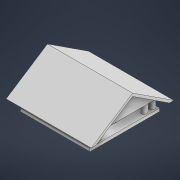
# Autodesk Inventor part: 110033226_ipt_15_房子屋頂
Saved by Autodesk Inventor 2022 (Build 260153000, 153)
## iProperties
Created: 2022-06-23
Part Number: 110033226_ipt_15_房子屋頂
Material: 一般
Document SubType Name: Modeling
Designer: User
Density: 1 g/cm^3
Appearance: 預設
Author: User
Autodesk Inventor part; units mm, degrees
ref_plane "YZ Plane" through (0, 0, 0) normal (1, 0, 0) x (0, 1, 0)
ref_plane "XZ Plane" through (0, 0, 0) normal (0, 1, 0) x (-1, 0, 0)
ref_plane "XY Plane" through (0, 0, 0) normal (0, 0, 1) x (1, 0, 0)
sketch "草圖1" plane through (0, 0, 0) normal (0, 1, 0) x (-1, 0, 0)
  line L0 (22.5, 22.5) -> (-22.5, 22.5)
  line L1 (-22.5, 22.5) -> (-22.5, -22.5)
  line L2 (-22.5, -22.5) -> (22.5, -22.5)
  line L3 (22.5, -22.5) -> (22.5, 22.5)
  circle A0 centre (20, 20) radius 1.7
  circle A1 centre (20, 15) radius 1.7
  circle A2 centre (20, 10) radius 1.7
  circle A3 centre (20, 5) radius 1.7
  circle A4 centre (20, 0) radius 1.7
  circle A5 centre (20, -5) radius 1.7
  circle A6 centre (20, -10) radius 1.7
  circle A7 centre (20, -15) radius 1.7
  circle A8 centre (20, -20) radius 1.7
  circle A9 centre (15, 20) radius 1.7
  circle A10 centre (15, 15) radius 1.7
  circle A11 centre (15, 10) radius 1.7
  circle A12 centre (15, 5) radius 1.7
  circle A13 centre (15, 0) radius 1.7
  circle A14 centre (15, -5) radius 1.7
  circle A15 centre (15, -10) radius 1.7
  circle A16 centre (15, -15) radius 1.7
  circle A17 centre (15, -20) radius 1.7
  circle A18 centre (10, 20) radius 1.7
  circle A19 centre (10, 15) radius 1.7
  circle A20 centre (10, 10) radius 1.7
  circle A21 centre (10, 5) radius 1.7
  circle A22 centre (10, 0) radius 1.7
  circle A23 centre (10, -5) radius 1.7
  circle A24 centre (10, -10) radius 1.7
  circle A25 centre (10, -15) radius 1.7
  circle A26 centre (10, -20) radius 1.7
  circle A27 centre (5, 20) radius 1.7
  circle A28 centre (5, 15) radius 1.7
  circle A29 centre (5, 10) radius 1.7
  circle A30 centre (5, 5) radius 1.7
  circle A31 centre (5, 0) radius 1.7
  circle A32 centre (5, -5) radius 1.7
  circle A33 centre (5, -10) radius 1.7
  circle A34 centre (5, -15) radius 1.7
  circle A35 centre (5, -20) radius 1.7
  circle A36 centre (0, 20) radius 1.7
  circle A37 centre (0, 15) radius 1.7
  circle A38 centre (0, 10) radius 1.7
  circle A39 centre (0, 5) radius 1.7
  circle A40 centre (0, 0) radius 1.7
  circle A41 centre (0, -5) radius 1.7
  circle A42 centre (0, -10) radius 1.7
  circle A43 centre (0, -15) radius 1.7
  circle A44 centre (0, -20) radius 1.7
  circle A45 centre (-5, 20) radius 1.7
  circle A46 centre (-5, 15) radius 1.7
  circle A47 centre (-5, 10) radius 1.7
  circle A48 centre (-5, 5) radius 1.7
  circle A49 centre (-5, 0) radius 1.7
  circle A50 centre (-5, -5) radius 1.7
  circle A51 centre (-5, -10) radius 1.7
  circle A52 centre (-5, -15) radius 1.7
  circle A53 centre (-5, -20) radius 1.7
  circle A54 centre (-10, 20) radius 1.7
  circle A55 centre (-10, 15) radius 1.7
  circle A56 centre (-10, 10) radius 1.7
  circle A57 centre (-10, 5) radius 1.7
  circle A58 centre (-10, 0) radius 1.7
  circle A59 centre (-10, -5) radius 1.7
  circle A60 centre (-10, -10) radius 1.7
  circle A61 centre (-10, -15) radius 1.7
  circle A62 centre (-10, -20) radius 1.7
  circle A63 centre (-15, 20) radius 1.7
  circle A64 centre (-15, 15) radius 1.7
  circle A65 centre (-15, 10) radius 1.7
  circle A66 centre (-15, 5) radius 1.7
  circle A67 centre (-15, 0) radius 1.7
  circle A68 centre (-15, -5) radius 1.7
  circle A69 centre (-15, -10) radius 1.7
  circle A70 centre (-15, -15) radius 1.7
  circle A71 centre (-15, -20) radius 1.7
  circle A72 centre (-20, 20) radius 1.7
  circle A73 centre (-20, 15) radius 1.7
  circle A74 centre (-20, 10) radius 1.7
  circle A75 centre (-20, 5) radius 1.7
  circle A76 centre (-20, 0) radius 1.7
  circle A77 centre (-20, -5) radius 1.7
  circle A78 centre (-20, -10) radius 1.7
  circle A79 centre (-20, -15) radius 1.7
  circle A80 centre (-20, -20) radius 1.7
  point P0 (0, 0)
  point P1 (22.5, 0)
  point P2 (0, -22.5)
  dimension "d0" = 45
  dimension "d1" = 45
  dimension "d2" = 3.4
  dimension "d3" = 2.5
  dimension "d4" = 2.5
  dimension "d7" = 5
  dimension "d10" = 5
  constraints: 81 centre point, 8 end point, 2 horizontal, 2 midpoint, 2 parallel, 1 horizontal alignment, 1 perpendicular, 1 vertical, 1 vertical alignment, 160 other
  measures "d0" distance of L2.end L1.end
  measures "d1" distance of L1.end L0.end
  measures "d2" diameter of A0
  measures "d3" distance from line of L3 A0.centre
  measures "d4" distance from line of L0 A0.centre
  measures "d7" distance of A0.centre A1.centre
  measures "d10" distance of A0.centre A9.centre
extrude "擠出1" add sketch "草圖1" along normal blind 6 contours A0 | A1 | A7 | A8 | A9 | A13 | A17 | A36 | A37 | A43 | A44 | A63 | A67 | A71 | A72 | A73 | A79 | A80
extrude "擠出2" add sketch "草圖1" against normal blind 2 contours L3 L2 L1 L0 | A0 | A1 | A2 | A3 | A4 | A5 | A6 | A7 | A8 | A9 | A10 | A11 | A12 | A13 | A14 | A15 | A16 | A17 | A18 | A19 | A20 | A21 | A22 | A23 | A24 | A25 | A26 | A27 | A28 | A29 | A30 | A31 | A32 | A33 | A34 | A35 | A36 | A37 | A38 | A39 | A40 | A41 | A42 | A43 | A44 | A45 | A46 | A47 | A48 | A49 | A50 | A51 | A52 | A53 | A54 | A55 | A56 | A57 | A58 | A59 | A60 | A61 | A62 | A63 | A64 | A65 | A66 | A67 | A68 | A69 | A70 | A71 | A72 | A73 | A74 | A75 | A76 | A77 | A78 | A79 | A80
sketch "草圖2" plane through (0, -2, 0) normal (0, -1, 0) x (1, 0, 0)
  circle A0 centre (20, 20) radius 1.7 projected
  circle A1 centre (20, 15) radius 1.7 projected
  circle A2 centre (15, 20) radius 1.7 projected
  line L0 (22.5, 22.5) -> (22.5, -22.5) projected
  line L1 (22.5, -22.5) -> (-22.5, -22.5) projected
  line L2 (-22.5, -22.5) -> (-22.5, 22.5) projected
  line L3 (-22.5, 22.5) -> (22.5, 22.5) projected
  circle A3 centre (20, 20) radius 1.7 projected
  circle A4 centre (-15, -20) radius 1.7 projected
  circle A5 centre (-15, 20) radius 1.7 projected
  circle A6 centre (-20, -15) radius 1.7 projected
  circle A7 centre (20, 15) radius 1.7 projected
  circle A8 centre (20, -20) radius 1.7 projected
  circle A9 centre (15, -20) radius 1.7 projected
  circle A10 centre (-20, -20) radius 1.7 projected
  circle A11 centre (-20, 20) radius 1.7 projected
  circle A12 centre (-20, 15) radius 1.7 projected
  circle A13 centre (15, 20) radius 1.7 projected
  circle A14 centre (20, -15) radius 1.7 projected
  circle A15 centre (5, 20) radius 1.7 projected
  circle A16 centre (0, 20) radius 1.7 projected
  circle A17 centre (-5, 20) radius 1.7 projected
  circle A18 centre (-10, 20) radius 1.7 projected
  circle A19 centre (-15, 15) radius 1.7 projected
  circle A20 centre (20, 0) radius 1.7 projected
  circle A21 centre (20, 5) radius 1.7 projected
  circle A22 centre (20, 10) radius 1.7 projected
  circle A23 centre (15, 10) radius 1.7 projected
  circle A24 centre (15, 5) radius 1.7 projected
  circle A25 centre (10, 5) radius 1.7 projected
  circle A26 centre (10, 10) radius 1.7 projected
  circle A27 centre (5, 10) radius 1.7 projected
  circle A28 centre (5, 5) radius 1.7 projected
  circle A29 centre (5, 0) radius 1.7 projected
  circle A30 centre (10, -5) radius 1.7 projected
  circle A31 centre (5, -5) radius 1.7 projected
  circle A32 centre (0, -5) radius 1.7 projected
  circle A33 centre (-5, -5) radius 1.7 projected
  circle A34 centre (0, -10) radius 1.7 projected
  circle A35 centre (-5, -10) radius 1.7 projected
  circle A36 centre (0, -15) radius 1.7 projected
  circle A37 centre (-5, -15) radius 1.7 projected
  circle A38 centre (5, -15) radius 1.7 projected
  circle A39 centre (10, -20) radius 1.7 projected
  circle A40 centre (5, -20) radius 1.7 projected
  circle A41 centre (0, -20) radius 1.7 projected
  circle A42 centre (-5, -20) radius 1.7 projected
  circle A43 centre (-10, -20) radius 1.7 projected
  circle A44 centre (-10, -15) radius 1.7 projected
  circle A45 centre (-15, -10) radius 1.7 projected
  circle A46 centre (-20, -10) radius 1.7 projected
  circle A47 centre (-20, -5) radius 1.7 projected
  circle A48 centre (-20, 0) radius 1.7 projected
  circle A49 centre (-20, 5) radius 1.7 projected
  circle A50 centre (-20, 10) radius 1.7 projected
  circle A51 centre (-15, 5) radius 1.7 projected
  circle A52 centre (-15, 0) radius 1.7 projected
  circle A53 centre (-15, -5) radius 1.7 projected
  circle A54 centre (-15, -15) radius 1.7 projected
  circle A55 centre (-5, 5) radius 1.7 projected
  circle A56 centre (0, 5) radius 1.7 projected
  circle A57 centre (-5, 0) radius 1.7 projected
  circle A58 centre (-5, 10) radius 1.7 projected
  circle A59 centre (-10, 10) radius 1.7 projected
  line L4 (-22.5, 22.5) -> (22.5, 22.5) projected
  circle A60 centre (10, 20) radius 1.7 projected
  circle A61 centre (-5, 15) radius 1.7 projected
  circle A62 centre (0, 10) radius 1.7 projected
  circle A63 centre (0, 15) radius 1.7 projected
  circle A64 centre (5, 15) radius 1.7 projected
  circle A65 centre (-10, 15) radius 1.7 projected
  circle A66 centre (10, 15) radius 1.7 projected
  circle A67 centre (15, 15) radius 1.7 projected
  circle A68 centre (15, -10) radius 1.7 projected
  circle A69 centre (10, -10) radius 1.7 projected
  circle A70 centre (10, -15) radius 1.7 projected
  circle A71 centre (15, -5) radius 1.7 projected
  circle A72 centre (15, 0) radius 1.7 projected
  circle A73 centre (10, 0) radius 1.7 projected
  circle A74 centre (5, -10) radius 1.7 projected
  circle A75 centre (20, -10) radius 1.7 projected
  circle A76 centre (20, -5) radius 1.7 projected
  circle A77 centre (15, -15) radius 1.7 projected
  circle A78 centre (-15, 10) radius 1.7 projected
  circle A79 centre (-10, -5) radius 1.7 projected
  circle A80 centre (-10, 5) radius 1.7 projected
  circle A81 centre (-10, 0) radius 1.7 projected
  circle A82 centre (-10, -10) radius 1.7 projected
  point P0 (0, 0)
extrude "擠出3" cut sketch "草圖2" against normal blind 1.5 contours A0 | A1 | A2 | A4 | A5 | A6 | A8 | A9 | A10 | A11 | A12 | A14 | A15 | A16 | A17 | A18 | A19 | A20 | A21 | A22 | A23 | A24 | A25 | A26 | A27 | A28 | A29 | A30 | A31 | A32 | A33 | A34 | A35 | A36 | A37 | A38 | A39 | A40 | A41 | A42 | A43 | A44 | A45 | A46 | A47 | A48 | A49 | A50 | A51 | A52 | A53 | A54 | A55 | A56 | A57 | A58 | A59 | A60 | A61 | A62 | A63 | A64 | A65 | A66 | A67 | A68 | A69 | A70 | A71 | A72 | A73 | A74 | A75 | A76 | A77 | A78 | A79 | A80 | A81 | A82
ref_plane "工作平面1" through (0, 0, -22.5) normal (-1, 0, 0) x (0, 0, 1)
sketch "草圖3" plane through (0, 0, -22.5) normal (-1, 0, 0) x (0, 0, 1)
  line L0 (44.2, 0) -> (45, 0) projected
  line L1 (45, 0) -> (45, -2) projected
  line L2 (45, -2) -> (44.2, -2) projected
  line L3 (44.2, -2) -> (44.2, -0.5) projected
  line L4 (44.2, -0.5) -> (40.8, -0.5) projected
  line L5 (40.8, -0.5) -> (40.8, -2) projected
  line L6 (40.8, -2) -> (39.2, -2) projected
  line L7 (39.2, -2) -> (39.2, -0.5) projected
  line L8 (39.2, -0.5) -> (35.8, -0.5) projected
  line L9 (35.8, -0.5) -> (35.8, -2) projected
  line L10 (35.8, -2) -> (34.2, -2) projected
  line L11 (34.2, -2) -> (34.2, -0.5) projected
  line L12 (34.2, -0.5) -> (30.8, -0.5) projected
  line L13 (30.8, -0.5) -> (30.8, -2) projected
  line L14 (30.8, -2) -> (29.2, -2) projected
  line L15 (29.2, -2) -> (29.2, -0.5) projected
  line L16 (29.2, -0.5) -> (25.8, -0.5) projected
  line L17 (25.8, -0.5) -> (25.8, -2) projected
  line L18 (25.8, -2) -> (19.2, -2) projected
  line L19 (19.2, -2) -> (19.2, -0.5) projected
  line L20 (19.2, -0.5) -> (15.8, -0.5) projected
  line L21 (15.8, -0.5) -> (15.8, -2) projected
  line L22 (15.8, -2) -> (14.2, -2) projected
  line L23 (14.2, -2) -> (14.2, -0.5) projected
  line L24 (14.2, -0.5) -> (10.8, -0.5) projected
  line L25 (10.8, -0.5) -> (10.8, -2) projected
  line L26 (10.8, -2) -> (9.2, -2) projected
  line L27 (9.2, -2) -> (9.2, -0.5) projected
  line L28 (9.2, -0.5) -> (5.8, -0.5) projected
  line L29 (5.8, -0.5) -> (5.8, -2) projected
  line L30 (5.8, -2) -> (4.2, -2) projected
  line L31 (4.2, -2) -> (4.2, -0.5) projected
  line L32 (4.2, -0.5) -> (0.8, -0.5) projected
  line L33 (0.8, -0.5) -> (0.8, -2) projected
  line L34 (0.8, -2) -> (0, -2) projected
  line L35 (0, -2) -> (0, 0) projected
  line L36 (0, 0) -> (0.8, 0) projected
  line L37 (0.8, 0) -> (0.8, 6) projected
  line L38 (0.8, 6) -> (4.2, 6) projected
  line L39 (4.2, 6) -> (4.2, 0) projected
  line L40 (4.2, 0) -> (5.8, 0) projected
  line L41 (5.8, 0) -> (5.8, 6) projected
  line L42 (5.8, 6) -> (9.2, 6) projected
  line L43 (9.2, 6) -> (9.2, 0) projected
  line L44 (9.2, 0) -> (35.8, 0) projected
  line L45 (35.8, 0) -> (35.8, 6) projected
  line L46 (35.8, 6) -> (39.2, 6) projected
  line L47 (39.2, 6) -> (39.2, 0) projected
  line L48 (39.2, 0) -> (40.8, 0) projected
  line L49 (40.8, 0) -> (40.8, 6) projected
  line L50 (40.8, 6) -> (44.2, 6) projected
  line L51 (44.2, 6) -> (44.2, 0) projected
  line L52 (22.5, 0) -> (22.5, 29.5043) construction
  line L53 (22.5, 0) -> (22.5, 22) construction
  line L54 (22.5, 22) -> (49.1305, 4.6205)
  line L55 (44.2, 6) -> (40.8, 6) projected
  line L56 (49.1305, 4.6205) -> (46.3139, 4.6205)
  line L57 (46.3139, 4.6205) -> (22.5, 20.1618)
  line L58 (22.5, 22) -> (-4.1305, 4.6205)
  line L59 (-1.3139, 4.6205) -> (22.5, 20.1618)
  line L60 (-4.1305, 4.6205) -> (-1.3139, 4.6205)
  line L61 (0.8, 6) -> (44.2, 6)
  dimension "d19" = 22
  constraints: 18 end point, 3 horizontal, 3 point on line, 2 symmetric about line, 1 parallel, 1 vertical
  measures "d19" distance of L52.start L53.end
extrude "擠出4" add sketch "草圖3" along normal mid plane 45 contours L50 L61 L46 L42 L38 L59 L57
extrude "擠出5" add sketch "草圖3" along normal mid plane 55 separate body contours L57 L59 L60 L58 L54 L56
